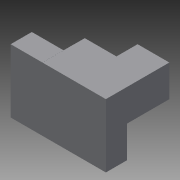
# Autodesk Inventor part: 128_0
Saved by Autodesk Inventor 2014 (Build 180170000, 170)
## iProperties
Created: 2017-04-22
Part Number: 128_0
Material: Generic
Document SubType Name: Modeling
Designer: Andy
Density: 1 g/cm^3
Appearance: Default
Author: Andy
Autodesk Inventor part; units mm, degrees
sketch "Sketch1" plane through (0, 0, 0) normal (0, 1, 0) x (-1, 0, 0)
  line L0 (0, 0) -> (30, 0)
  line L1 (30, 0) -> (30, -20)
  line L2 (30, -20) -> (0, -20)
  line L3 (0, -20) -> (0, 0)
  line L4 (0, 0) -> (10, 0)
  line L5 (10, 0) -> (10, -10)
  line L6 (10, -10) -> (0, -10)
  line L7 (0, -10) -> (0, 0)
  line L8 (10, 0) -> (20, 0)
  line L9 (20, 0) -> (20, -10)
  line L10 (20, -10) -> (10, -10)
  line L11 (10, -10) -> (10, 0)
  line L12 (20, 0) -> (30, 0)
  line L13 (30, 0) -> (30, -10)
  line L14 (30, -10) -> (20, -10)
  line L15 (20, -10) -> (20, 0)
  line L16 (0, -10) -> (10, -10)
  line L17 (10, -10) -> (10, -20)
  line L18 (10, -20) -> (0, -20)
  line L19 (0, -20) -> (0, -10)
  line L20 (10, -10) -> (20, -10)
  line L21 (20, -10) -> (20, -20)
  line L22 (20, -20) -> (10, -20)
  line L23 (10, -20) -> (10, -10)
  line L24 (20, -10) -> (30, -10)
  line L25 (30, -10) -> (30, -20)
  line L26 (30, -20) -> (20, -20)
  line L27 (20, -20) -> (20, -10)
  dimension "d0" = 30
  dimension "d1" = 20
  dimension "d2" = 10
  dimension "d3" = 10
  constraints: 56 end point, 14 parallel, 7 horizontal, 7 perpendicular, 2 point on line, 1 midpoint
  measures "d0" distance of L1.end L2.end
  measures "d1" distance of L0.end L1.end
  measures "d2" distance of L5.end L6.end
  measures "d3" distance of L9.end L10.end
extrude "Extrusion1" add sketch "Sketch1" along normal blind 20 contours L10 L21 L2 L17
ref_plane "Work Plane2" through (-10, 0, -10) normal (0, 1, 0) x (0, 0, -1)
sketch "Sketch2" plane through (-10, 0, -10) normal (0, 1, 0) x (0, 0, -1)
  line L0 (0, 0) -> (-10, 0)
  line L1 (-10, 0) -> (-10, 10)
  line L2 (-10, 10) -> (0, 10)
  line L3 (0, 10) -> (0, 0)
  point P0 (-10, -10)
  dimension "d6" = 10
  dimension "d7" = 10
  constraints: 8 end point, 2 parallel, 1 horizontal, 1 perpendicular
  measures "d6" distance of L1.end L2.end
  measures "d7" distance of L0.end L1.end
extrude "Extrusion2" add sketch "Sketch2" along normal blind 6.67
ref_plane "Work Plane3" through (-10, 0, -10) normal (0, 1, 0) x (0, 0, -1)
sketch "Sketch3" plane through (-10, 0, -10) normal (0, 1, 0) x (0, 0, -1)
  line L0 (-10, -0.023) -> (10, -0.023)
  line L1 (10, -0.023) -> (10, -10.023)
  line L2 (10, -10.023) -> (-10, -10.023)
  line L3 (-10, -10.023) -> (-10, -0.023)
  point P0 (-10, -10)
  dimension "d10" = 20
  dimension "d11" = 10
  constraints: 8 end point, 2 parallel, 1 horizontal, 1 perpendicular
  measures "d10" distance of L1.end L2.end
  measures "d11" distance of L0.end L1.end
extrude "Extrusion3" add sketch "Sketch3" along normal blind 13.33
ref_plane "Work Plane4" through (-10, 0, -10) normal (0, -1, 0) x (1, 0, 0)
sketch "Sketch4" plane through (-10, 0, -10) normal (0, -1, 0) x (1, 0, 0)
  line L0 (10, 10) -> (20, 10)
  line L1 (20, 10) -> (20, 0)
  line L2 (20, 0) -> (10, 0)
  line L3 (10, 0) -> (10, 10)
  dimension "d14" = 10
  constraints: 8 end point, 2 parallel, 1 horizontal, 1 perpendicular
  measures "d14" distance of L1.end L2.end
extrude "Extrusion4" add sketch "Sketch4" against normal blind 20
ref_plane "Work Plane5" through (-10, 0, -10) normal (0, -1, 0) x (1, 0, 0)
sketch "Sketch5" plane through (-10, 0, -10) normal (0, -1, 0) x (1, 0, 0)
  line L0 (10.023, 0) -> (20, 0)
  line L1 (20, 0) -> (20, -10)
  line L2 (20, -10) -> (10.023, -10)
  line L3 (10.023, -10) -> (10.023, 0)
  point P0 (10, 10)
  constraints: 8 end point, 2 parallel, 1 horizontal, 1 perpendicular
extrude "Extrusion5" add sketch "Sketch5" against normal blind 6.67
body "Solid1"
